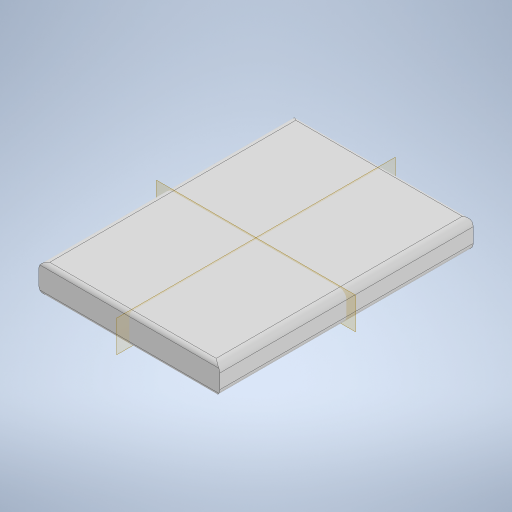
# Autodesk Inventor part: Battery_402535
Saved by Autodesk Inventor 2023 (Build 270158000, 158)
## iProperties
Created: 2023-03-12
Part Number: Battery_402535
Material: Generic
Document SubType Name: Modeling
Designer: nigel
Density: 1 g/cm^3
Appearance: Default
Author: nigel
Autodesk Inventor part; units mm, degrees
ref_plane "YZ Plane" through (0, 0, 0) normal (1, 0, 0) x (0, 1, 0)
ref_plane "XZ Plane" through (0, 0, 0) normal (0, 1, 0) x (-1, 0, 0)
ref_plane "XY Plane" through (0, 0, 0) normal (0, 0, 1) x (1, 0, 0)
sketch "Sketch1" plane through (0, 0, 0) normal (0, 1, 0) x (-1, 0, 0)
  line L0 (0, 0) -> (-25, 0)
  line L1 (-25, 0) -> (-25, -35)
  line L2 (-25, -35) -> (0, -35)
  line L3 (0, -35) -> (0, 0)
  dimension "d0" = 25
  dimension "d1" = 35
  constraints: 8 end point, 2 parallel, 1 horizontal, 1 perpendicular
  measures "d0" distance of L1.end L2.end
  measures "d1" distance of L2.end L0.start
extrude "Extrusion1" add sketch "Sketch1" along normal blind 4
fillet "Fillet1" radius 1 4 edges at (0, 4, -17.5) (0, 0, -17.5) (25, 4, -17.5) (25, 0, -17.5)
fillet "Fillet1" radius 0.5 4 edges at (12.5, 4, -35) (12.5, 0, -35) (12.5, 4, 0) (12.5, 0, 0)
ref_plane "Work Plane1" through (12.5, 1, -35) normal (1, 0, 0) x (0, 0, -1)
ref_plane "Work Plane2" through (0.134, 3.5, -17.5) normal (0, 0, 1) x (1, 0, 0)
body "Solid1"
